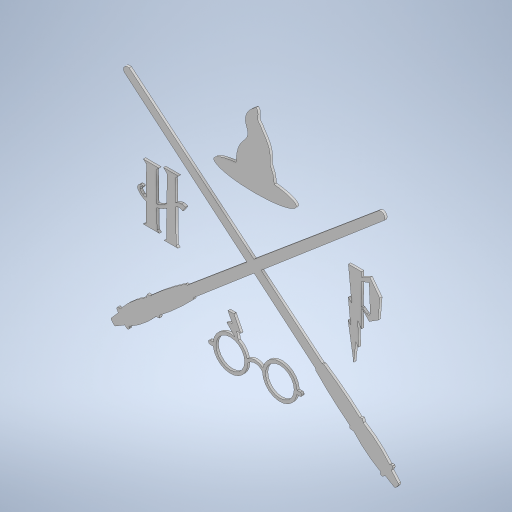
# Autodesk Inventor part: HP cross sign peices
Saved by Autodesk Inventor 2024 (Build 280153000, 153)
## iProperties
Created: 2023-06-06
Part Number: HP cross sign peices
Material: Generic
Document SubType Name: Modeling
Designer: newic
Density: 1 g/cm^3
Appearance: Default
Author: newic
Autodesk Inventor part; units mm, degrees
ref_plane "YZ Plane" through (0, 0, 0) normal (1, 0, 0) x (0, 1, 0)
ref_plane "XZ Plane" through (0, 0, 0) normal (0, 1, 0) x (-1, 0, 0)
ref_plane "XY Plane" through (0, 0, 0) normal (0, 0, 1) x (1, 0, 0)
sketch "Sketch1" plane through (0, 0, 0) normal (0, 0, 1) x (1, 0, 0)
  line L0 (50.8, 0) -> (355.6, 0)
  line L1 (406.4, 50.8) -> (406.4, 355.6)
  line L2 (355.6, 406.4) -> (50.8, 406.4)
  line L3 (0, 355.6) -> (0, 50.8)
  line L4 (-614.419348, 544.235047) -> (888.726493, 544.235047) construction
  line L5 (888.726493, 544.235047) -> (888.726493, -583.124441) construction
  line L6 (888.726493, -583.124441) -> (-614.419348, -583.124441) construction
  line L7 (-614.419348, -583.124441) -> (-614.419348, 544.235047) construction
  line L8 (6.363818, 43.79595) -> (9.763503, 39.85729)
  line L9 (12.196347, 39.474947) -> (24.470176, 46.948616)
  line L10 (24.470176, 46.948616) -> (27.553601, 44.522314)
  line L11 (29.72239, 44.392306) -> (30.075019, 44.607026)
  line L12 (30.938043, 46.672901) -> (30.552839, 48.300319)
  arc A0 (30.552839, 48.300319) -> (68.057484, 78.865401) centre (-37.470935, 170.060789) ccw
  arc A1 (68.057484, 78.865401) -> (72.898915, 79.406809) centre (69.41099, 88.679409) ccw
  arc A2 (72.898915, 79.406809) -> (72.898915, 82.717894) centre (67.457972, 81.062352) ccw
  arc A3 (72.898915, 82.717894) -> (119.938243, 125.239443) centre (-186.405748, 416.852181) ccw
  arc A4 (119.938243, 125.239443) -> (119.938243, 127.366674) centre (115.200777, 126.303058) ccw
  arc A5 (383.588883, 351.74213) -> (376.499139, 359.921937) centre (378.691736, 354.659966) ccw
  line L13 (6.368301, 46.290626) -> (15.835186, 57.178989)
  line L14 (15.835186, 57.178989) -> (13.961148, 60.626079)
  line L15 (14.197196, 62.7859) -> (14.468084, 63.097463)
  line L16 (16.64955, 63.601304) -> (18.189169, 62.948274)
  arc A6 (54.618428, 94.787427) -> (18.189169, 62.948274) centre (126.797058, -24.556995) ccw
  arc A7 (55.965181, 99.469183) -> (54.618428, 94.787427) centre (64.52036, 94.473621) ccw
  arc A8 (59.229243, 98.913144) -> (55.965181, 99.469183) centre (56.683501, 93.827491) ccw
  arc A9 (109.046352, 138.143695) -> (59.229243, 98.913144) centre (345.072656, -212.820994) ccw
  arc A10 (111.143373, 137.786464) -> (109.046352, 138.143695) centre (109.299288, 133.294893) ccw
  arc A11 (383.535154, 351.737832) -> (376.60786, 360.012951) centre (378.661869, 354.695351) ccw
  arc A12 (27.553601, 44.522314) -> (29.72239, 44.392306) centre (28.731635, 46.019399) ccw
  arc A13 (9.763503, 39.85729) -> (12.196347, 39.474947) centre (11.205592, 41.10204) ccw
  arc A14 (6.368301, 46.290626) -> (6.363818, 43.79595) centre (7.805907, 45.0407) ccw
  arc A15 (14.197196, 62.7859) -> (13.961148, 60.626079) centre (15.634801, 61.535974) ccw
  arc A16 (16.64955, 63.601304) -> (14.468084, 63.097463) centre (15.90569, 61.847537) ccw
  arc A17 (30.075019, 44.607026) -> (30.938043, 46.672901) centre (29.084264, 46.234118) ccw
  line L17 (399.519466, 39.849724) -> (402.80794, 43.881702)
  line L18 (402.762015, 46.343978) -> (393.27056, 57.133552)
  line L19 (393.27056, 57.133552) -> (395.12457, 60.591456)
  line L20 (394.875997, 62.749871) -> (394.603305, 63.059857)
  line L21 (392.418953, 63.551035) -> (390.883149, 62.889085)
  arc A18 (390.883149, 62.889085) -> (354.269806, 94.516378) centre (282.784699, -25.244739) ccw
  arc A19 (354.269806, 94.516378) -> (352.895917, 99.190243) centre (344.369861, 94.145137) ccw
  arc A20 (352.895917, 99.190243) -> (349.635135, 98.615279) centre (352.210336, 93.544479) ccw
  arc A21 (349.635135, 98.615279) -> (299.591291, 137.556184) centre (65.604881, -214.771773) ccw
  arc A22 (299.591291, 137.556184) -> (297.496377, 137.186795) centre (299.366486, 132.705996) ccw
  arc A23 (340.923339, 78.516662) -> (378.604658, 48.169656) centre (445.920964, 170.322678) ccw
  line L22 (384.69506, 46.853261) -> (381.625761, 44.409113)
  line L23 (397.061911, 39.420944) -> (384.69506, 46.853261)
  line L24 (379.457764, 44.266526) -> (379.103895, 44.479196)
  line L25 (378.228901, 46.54003) -> (378.604658, 48.169656)
  arc A24 (336.078849, 79.029976) -> (340.923339, 78.516662) centre (339.512925, 88.322652) ccw
  arc A25 (336.059641, 82.341005) -> (336.078849, 79.029976) centre (341.510096, 80.717053) ccw
  arc A26 (288.77444, 124.588966) -> (336.059641, 82.341005) centre (593.42165, 417.973879) ccw
  arc A27 (288.7621, 126.716161) -> (288.77444, 124.588966) centre (293.505656, 125.680045) ccw
  arc A28 (30.856483, 357.779219) -> (23.814309, 349.558422) centre (28.694447, 352.504618) ccw
  arc A29 (395.12457, 60.591456) -> (394.875997, 62.749871) centre (393.445666, 61.491627) ccw
  arc A30 (402.80794, 43.881702) -> (402.762015, 46.343978) centre (401.331684, 45.085734) ccw
  arc A31 (397.061911, 39.420944) -> (399.519466, 39.849724) centre (398.04321, 41.053756) ccw
  arc A32 (379.457764, 44.266526) -> (381.625761, 44.409113) centre (380.439063, 45.899338) ccw
  arc A33 (378.228901, 46.54003) -> (379.103895, 44.479196) centre (380.085194, 46.112009) ccw
  arc A34 (394.603305, 63.059857) -> (392.418953, 63.551035) centre (393.172975, 61.801613) ccw
  line L26 (401.147574, 41.845938) -> (389.574066, 107.482563) construction
  line L27 (321.553196, 108.082514) -> (389.468279, 108.082514) construction
  circle A35 centre (170.75121, 85.859958) radius 19.77729
  circle A36 centre (239.095683, 86.367375) radius 19.77729
  arc A37 (215.16651, 86.367375) -> (194.675003, 86.367375) centre (204.920756, 78.710251) ccw
  arc A38 (215.689784, 91.344244) -> (194.061536, 91.266807) centre (204.920756, 78.710251) ccw
  line L28 (269.404649, 85.988013) -> (269.404649, 84.655093)
  line L29 (140.68774, 84.655093) -> (140.68774, 85.988013)
  line L30 (267.499649, 82.750093) -> (262.749871, 82.750093)
  line L31 (147.024978, 82.750093) -> (142.59274, 82.750093)
  line L32 (142.59274, 87.893013) -> (146.908559, 87.893013)
  line L33 (262.976172, 87.893013) -> (267.499649, 87.893013)
  arc A39 (142.59274, 87.893013) -> (140.68774, 85.988013) centre (142.59274, 85.988013) ccw
  arc A40 (140.68774, 84.655093) -> (142.59274, 82.750093) centre (142.59274, 84.655093) ccw
  arc A41 (267.499649, 82.750093) -> (269.404649, 84.655093) centre (267.499649, 84.655093) ccw
  arc A42 (269.404649, 85.988013) -> (267.499649, 87.893013) centre (267.499649, 85.988013) ccw
  line L34 (176.805781, 109.010498) -> (165.933338, 120.455956)
  line L35 (173.368384, 123.688879) -> (167.378721, 135.467811)
  line L36 (167.60513, 135.836942) -> (175.47758, 135.836942)
  line L37 (175.703989, 135.698072) -> (185.025768, 117.366391)
  line L38 (184.799359, 116.99726) -> (179.672528, 116.99726)
  line L39 (179.426041, 116.681942) -> (181.815289, 107.077674)
  line L40 (166.035192, 120.871189) -> (173.224277, 123.333452)
  arc A43 (166.035192, 120.871189) -> (165.933338, 120.455956) centre (166.117494, 120.630892) ccw
  arc A44 (179.672528, 116.99726) -> (179.426041, 116.681942) centre (179.672528, 116.74326) ccw
  arc A45 (173.224277, 123.333452) -> (173.368384, 123.688879) centre (173.141975, 123.573749) ccw
  arc A46 (184.799359, 116.99726) -> (185.025768, 117.366391) centre (184.799359, 117.25126) ccw
  arc A47 (175.703989, 135.698072) -> (175.47758, 135.836942) centre (175.47758, 135.582942) ccw
  arc A48 (167.60513, 135.836942) -> (167.378721, 135.467811) centre (167.60513, 135.582942) ccw
  line L41 (79.178486, 175.528718) -> (98.216612, 175.528718)
  line L42 (98.216612, 175.528718) -> (95.757723, 177.666599)
  line L43 (79.178486, 175.528718) -> (82.322522, 178.515348)
  line L44 (83.401566, 257.118075) -> (78.414715, 262.36775)
  line L45 (78.414715, 262.36775) -> (99.063012, 262.36775)
  line L46 (99.063012, 262.36775) -> (94.659721, 258.18491)
  arc A49 (104.876764, 223.458347) -> (95.13125, 223.606943) centre (99.925457, 218.381083) ccw
  arc A50 (103.246066, 231.262323) -> (95.066939, 228.322925) centre (103.717194, 217.10211) ccw
  arc A51 (109.046352, 230.12172) -> (103.246066, 231.262323) centre (102.604733, 212.682614) ccw
  line L47 (104.876764, 223.458347) -> (109.046352, 230.12172)
  arc A52 (68.934077, 213.993149) -> (82.910758, 221.36528) centre (58.833092, 250.078534) ccw
  arc A53 (69.00456, 209.415023) -> (82.833167, 215.713199) centre (58.833092, 250.078534) ccw
  line L48 (68.309171, 254.582837) -> (71.925781, 258.465439)
  line L49 (71.925781, 258.465439) -> (50.439964, 258.597904)
  line L50 (50.439964, 258.597904) -> (54.618428, 254.705701)
  line L51 (54.180223, 183.62886) -> (50.217049, 180.722268)
  line L52 (50.217049, 180.722268) -> (72.473079, 180.585054)
  line L53 (72.473079, 180.585054) -> (69.41099, 183.016097)
  arc A54 (49.876677, 216.000145) -> (54.372837, 214.870815) centre (53.327561, 220.224164) ccw
  arc A55 (46.111078, 220.518863) -> (49.876677, 216.000145) centre (54.303486, 223.517512) ccw
  arc A56 (46.539208, 223.606943) -> (46.111078, 220.518863) centre (48.44907, 221.768443) ccw
  arc A57 (49.303504, 223.746898) -> (46.539208, 223.606943) centre (48.03713, 221.390233) ccw
  arc A58 (50.495329, 225.859285) -> (49.303504, 223.746898) centre (51.842309, 223.706896) ccw
  arc A59 (50.495329, 225.859285) -> (46.539208, 226.329877) centre (48.121838, 222.770318) ccw
  arc A60 (46.539208, 226.329877) -> (42.629235, 222.901423) centre (48.780718, 219.829765) ccw
  arc A61 (42.629235, 222.901423) -> (44.2476, 216.93411) centre (48.159437, 221.198131) ccw
  arc A62 (44.2476, 216.93411) -> (54.343434, 210.101637) centre (58.241765, 226.737074) ccw
  ellipse E0 centre (204.861319, 307.520258) end of major axis (261.987782, 307.520258) minor radius 12.590113 (178.424158, 318.681034) -> (231.29848, 318.681034) ccw
  spline S0 degree 4 poles (178.424158, 318.681034) (179.286467, 323.908779) (178.746893, 329.903111) (181.705459, 341.161729) (188.374596, 349.276888) (192.595103, 353.973206) (195.221019, 358.516301) (195.296154, 364.688161) (192.664089, 369.267258) (190.583011, 375.858216) (192.831333, 385.567134) (196.944916, 391.686323) (204.688734, 396.950297) (206.423918, 398.265857) knots 0 0 0 0 0 0.21195074 0.29434202 0.37160428 0.44319933 0.51142961 0.58048484 0.65260868 0.72741885 0.80713657 1 1 1 1 1
  spline S1 degree 4 poles (231.29848, 318.681034) (230.812293, 323.383734) (230.310579, 325.948758) (229.967534, 332.297352) (225.164417, 337.865291) (225.794617, 343.609489) (225.873041, 348.569917) (225.596308, 353.136069) (224.268791, 359.169129) (219.906128, 368.536889) (215.480963, 372.873287) (212.6971, 379.704121) (210.084613, 381.955148) (208.358926, 383.728321) (209.16421, 389.030713) (208.726826, 393.481301) (209.350832, 395.663281) (206.387951, 397.79334) (206.423918, 398.265857) knots 0 0 0 0 0 0.14868292 0.20666124 0.26562711 0.32344479 0.38253037 0.44758088 0.5167693 0.58902303 0.65607066 0.71151816 0.76312054 0.81115478 0.85814688 0.90611656 1 1 1 1 1
  line L54 (344.02064, 186.46558) -> (341.227275, 160.617354)
  line L55 (341.227275, 160.617354) -> (333.409452, 207.367115)
  line L56 (333.409452, 207.367115) -> (336.992659, 203.165326)
  line L57 (336.992659, 203.165326) -> (333.673251, 234.780696)
  line L58 (333.673251, 234.780696) -> (338.519545, 230.387183)
  line L59 (338.519545, 230.387183) -> (333.891431, 274.467202)
  line L60 (333.891431, 274.467202) -> (352.210336, 274.467202)
  line L61 (352.210336, 274.467202) -> (352.210336, 267.640425)
  line L62 (352.210336, 267.640425) -> (363.576578, 273.420233)
  line L63 (363.576578, 273.420233) -> (377.295, 255.343095)
  line L64 (377.295, 255.343095) -> (374.999674, 227.922054)
  line L65 (374.999674, 227.922054) -> (362.58525, 220.224164)
  line L66 (362.58525, 220.224164) -> (353.775486, 229.691563)
  line L67 (353.775486, 229.691563) -> (351.68678, 229.917285)
  line L68 (351.68678, 229.917285) -> (352.014132, 205.911995)
  line L69 (352.014132, 205.911995) -> (346.906345, 213.168267)
  line L70 (346.906345, 213.168267) -> (347.892244, 181.925607)
  line L71 (347.892244, 181.925607) -> (344.02064, 186.46558)
  line L72 (351.658839, 231.966214) -> (353.63723, 231.752414)
  line L73 (353.63723, 231.752414) -> (359.583199, 227.519206)
  line L74 (359.583199, 227.519206) -> (362.173085, 227.109648)
  line L75 (362.173085, 227.109648) -> (364.249648, 230.605551)
  line L76 (364.249648, 230.605551) -> (362.58525, 266.672272)
  line L77 (362.58525, 266.672272) -> (352.014132, 262.742303)
  line L78 (352.014132, 262.742303) -> (351.658839, 231.966214)
  line L79 (94.659721, 258.18491) -> (95.066939, 228.322925)
  line L80 (95.13125, 223.606943) -> (95.757723, 177.666599)
  line L81 (82.322522, 178.515348) -> (82.833167, 215.713199)
  line L82 (82.910758, 221.36528) -> (83.401566, 257.118075)
  line L83 (69.41099, 183.016097) -> (69.00456, 209.415023)
  line L84 (68.934077, 213.993149) -> (68.309171, 254.582837)
  line L85 (54.618428, 254.705701) -> (54.372837, 214.870815)
  line L86 (54.343434, 210.101637) -> (54.180223, 183.62886)
  line L87 (288.7621, 126.716161) -> (203.469206, 198.4543)
  line L88 (193.5656, 206.784024) -> (23.814309, 349.558422)
  line L89 (111.143373, 137.786464) -> (193.5656, 206.784024)
  line L90 (203.409935, 215.024946) -> (376.60786, 360.012951)
  line L91 (297.496377, 137.186795) -> (213.313238, 206.831897)
  line L92 (203.409935, 215.024946) -> (30.747236, 357.8696)
  line L93 (119.938243, 127.366674) -> (203.469206, 198.4543)
  line L94 (213.313238, 206.831897) -> (383.588883, 351.74213)
  arc A63 (147.024978, 82.750093) -> (194.675003, 86.367375) centre (170.75121, 85.859958) ccw
  arc A64 (194.061536, 91.266807) -> (181.815289, 107.077674) centre (170.75121, 85.859958) ccw
  arc A65 (176.805781, 109.010498) -> (146.908559, 87.893013) centre (170.75121, 85.859958) ccw
  arc A66 (215.16651, 86.367375) -> (262.749871, 82.750093) centre (239.095683, 86.367375) ccw
  arc A67 (262.976172, 87.893013) -> (215.689784, 91.344244) centre (239.095683, 86.367375) ccw
  arc A68 (0, 50.8) -> (50.8, 0) centre (50.8, 50.8) ccw
  arc A69 (355.6, 0) -> (406.4, 50.8) centre (355.6, 50.8) ccw
  arc A70 (406.4, 355.6) -> (355.6, 406.4) centre (355.6, 355.6) ccw
  arc A71 (50.8, 406.4) -> (0, 355.6) centre (50.8, 355.6) ccw
  point P0 (0, 0)
  point P1 (406.4, 406.4)
  point P2 (406.4, 0)
  point P3 (0, 406.4)
  point P4 (0, 51.168666)
  point P5 (10.817977, 38.635643)
  point P6 (28.59287, 43.704529)
  point P7 (31.256714, 45.326573)
  point P8 (5.347622, 45.116689)
  point P9 (13.329503, 61.787921)
  point P10 (15.375857, 64.141541)
  point P11 (179.198193, 326.398969)
  point P12 (180.643488, 334.841283)
  point P13 (184.294349, 343.588045)
  point P14 (188.857454, 349.748318)
  point P15 (192.58381, 354.387156)
  point P16 (194.713184, 358.874049)
  point P17 (194.789154, 364.197382)
  point P18 (192.963469, 369.215634)
  point P19 (191.366125, 375.527158)
  point P20 (192.431013, 382.448126)
  point P21 (195.777407, 388.760699)
  point P22 (202.089525, 394.996718)
  point P23 (230.558885, 324.790873)
  point P24 (229.864918, 328.854993)
  point P25 (228.278944, 333.514177)
  point P26 (225.999136, 338.173488)
  point P27 (225.701673, 343.625386)
  point P28 (225.800615, 348.383168)
  point P29 (225.50309, 352.546274)
  point P30 (224.115391, 358.494162)
  point P31 (219.555898, 368.011288)
  point P32 (215.095419, 374.554337)
  point P33 (211.923531, 380.006823)
  point P34 (210.040123, 382.088572)
  point P35 (208.949651, 383.971886)
  point P36 (208.949495, 388.927986)
  point P37 (208.949275, 392.793548)
  point P38 (208.651649, 395.073014)
  point P39 (207.164723, 397.25383)
  dimension "d0" = 406.4
  dimension "d1" = 406.4
  dimension "d37" = 1.905
  dimension "d38" = 1.905
  dimension "d40" = 1.905
  dimension "d41" = 1.905
  dimension "d43" = 1.905
  dimension "d44" = 1.905
  dimension "d45" = 1.905
  dimension "d46" = 1.905
  dimension "d62" = 3.81
  dimension "d69" = 1.905
  dimension "d73" = 0.254
  dimension "d80" = 50.8
  constraints: 182 end point, 141 point on circle, 72 centre point, 52 tangent, 27 point on line, 15 equal radius, 15 parallel, 9 horizontal, 7 perpendicular, 2 coincident, 41 other
  measures "d0" distance of point (0, 406.4) point (406.4, 406.4)
  measures "d1" distance of point (406.4, 406.4) point (406.4, 0)
  measures "d37" radius of A12
  measures "d38" radius of A13
  measures "d40" radius of A14
  measures "d41" radius of A15
  measures "d43" radius of A29
  measures "d44" radius of A30
  measures "d45" radius of A31
  measures "d46" radius of A32
  measures "d62" radial gap between concentric circles of A37 A38
  measures "d69" radius of A39
  measures "d73" radius of A43
  measures "d80" radius of A68
sketch "Sketch1 outline for Extrusion1" plane through (0, 0, 0) normal (0, 0, 1) x (1, 0, 0)
  arc A0 (267.499649, 82.750093) -> (269.404649, 84.655093) centre (267.499649, 84.655093) ccw
  line L0 (262.749871, 82.750093) -> (267.499649, 82.750093)
  line L1 (269.404649, 84.655093) -> (269.404649, 85.988013)
  arc A1 (215.16651, 86.367375) -> (262.749871, 82.750093) centre (239.095683, 86.367375) ccw
  arc A2 (269.404649, 85.988013) -> (267.499649, 87.893013) centre (267.499649, 85.988013) ccw
  arc A3 (194.675003, 86.367375) -> (215.16651, 86.367375) centre (204.920756, 78.710251) cw
  line L2 (267.499649, 87.893013) -> (262.976172, 87.893013)
  arc A4 (147.024978, 82.750093) -> (194.675003, 86.367375) centre (170.75121, 85.859958) ccw
  arc A5 (262.976172, 87.893013) -> (215.689784, 91.344244) centre (239.095683, 86.367375) ccw
  line L3 (142.59274, 82.750093) -> (147.024978, 82.750093)
  arc A6 (215.689784, 91.344244) -> (194.061536, 91.266807) centre (204.920756, 78.710251) ccw
  arc A7 (140.68774, 84.655093) -> (142.59274, 82.750093) centre (142.59274, 84.655093) ccw
  arc A8 (194.061536, 91.266807) -> (181.815289, 107.077674) centre (170.75121, 85.859958) ccw
  line L4 (140.68774, 85.988013) -> (140.68774, 84.655093)
  line L5 (181.815289, 107.077674) -> (179.426041, 116.681942)
  arc A9 (142.59274, 87.893013) -> (140.68774, 85.988013) centre (142.59274, 85.988013) ccw
  arc A10 (179.426041, 116.681942) -> (179.672528, 116.99726) centre (179.672528, 116.74326) cw
  line L6 (146.908559, 87.893013) -> (142.59274, 87.893013)
  line L7 (179.672528, 116.99726) -> (184.799359, 116.99726)
  arc A11 (176.805781, 109.010498) -> (146.908559, 87.893013) centre (170.75121, 85.859958) ccw
  arc A12 (184.799359, 116.99726) -> (185.025768, 117.366391) centre (184.799359, 117.25126) ccw
  line L8 (165.933338, 120.455956) -> (176.805781, 109.010498)
  line L9 (185.025768, 117.366391) -> (175.703989, 135.698072)
  arc A13 (166.035192, 120.871189) -> (165.933338, 120.455956) centre (166.117494, 120.630892) ccw
  arc A14 (175.703989, 135.698072) -> (175.47758, 135.836942) centre (175.47758, 135.582942) ccw
  line L10 (173.224277, 123.333452) -> (166.035192, 120.871189)
  line L11 (175.47758, 135.836942) -> (167.60513, 135.836942)
  arc A15 (173.368384, 123.688879) -> (173.224277, 123.333452) centre (173.141975, 123.573749) cw
  arc A16 (167.60513, 135.836942) -> (167.378721, 135.467811) centre (167.60513, 135.582942) ccw
  line L12 (167.378721, 135.467811) -> (173.368384, 123.688879)
  circle A17 centre (170.75121, 85.859958) radius 19.77729
  circle A18 centre (239.095683, 86.367375) radius 19.77729
  line L13 (344.02064, 186.46558) -> (347.892244, 181.925607)
  line L14 (341.227275, 160.617354) -> (344.02064, 186.46558)
  line L15 (347.892244, 181.925607) -> (346.906345, 213.168267)
  line L16 (333.409452, 207.367115) -> (341.227275, 160.617354)
  line L17 (346.906345, 213.168267) -> (352.014132, 205.911995)
  line L18 (336.992659, 203.165326) -> (333.409452, 207.367115)
  line L19 (352.014132, 205.911995) -> (351.68678, 229.917285)
  line L20 (333.673251, 234.780696) -> (336.992659, 203.165326)
  line L21 (351.68678, 229.917285) -> (353.775486, 229.691563)
  line L22 (338.519545, 230.387183) -> (333.673251, 234.780696)
  line L23 (353.775486, 229.691563) -> (362.58525, 220.224164)
  line L24 (333.891431, 274.467202) -> (338.519545, 230.387183)
  line L25 (362.58525, 220.224164) -> (374.999674, 227.922054)
  line L26 (352.210336, 274.467202) -> (333.891431, 274.467202)
  line L27 (374.999674, 227.922054) -> (377.295, 255.343095)
  line L28 (352.210336, 267.640425) -> (352.210336, 274.467202)
  line L29 (377.295, 255.343095) -> (363.576578, 273.420233)
  line L30 (363.576578, 273.420233) -> (352.210336, 267.640425)
  line L31 (351.658839, 231.966214) -> (352.014132, 262.742303)
  line L32 (353.63723, 231.752414) -> (351.658839, 231.966214)
  line L33 (359.583199, 227.519206) -> (353.63723, 231.752414)
  line L34 (362.173085, 227.109648) -> (359.583199, 227.519206)
  line L35 (364.249648, 230.605551) -> (362.173085, 227.109648)
  line L36 (362.58525, 266.672272) -> (364.249648, 230.605551)
  line L37 (352.014132, 262.742303) -> (362.58525, 266.672272)
  spline S0 degree 2 poles (178.424158, 318.681034) (116.307715, 311.534236) (160.584517, 299.56482) (204.861319, 287.595404) (249.138121, 299.56482) (293.414923, 311.534236) (231.29848, 318.681034) knots 0 0 0 0.33333333 0.33333333 0.66666667 0.66666667 1 1 1 weights 1 0.6318798 1 0.6318798 1 0.6318798 1
  spline S1 degree 4 poles (178.424158, 318.681034) (179.286467, 323.908779) (178.746893, 329.903111) (181.705459, 341.161729) (188.374596, 349.276888) (192.595103, 353.973206) (195.221019, 358.516301) (195.296154, 364.688161) (192.664089, 369.267258) (190.583011, 375.858216) (192.831333, 385.567134) (196.944916, 391.686323) (204.688734, 396.950297) (206.423918, 398.265857) knots 0 0 0 0 0 0.21195074 0.29434202 0.37160428 0.44319933 0.51142961 0.58048484 0.65260868 0.72741885 0.80713657 1 1 1 1 1
  spline S2 degree 4 poles (231.29848, 318.681034) (230.812293, 323.383734) (230.310579, 325.948758) (229.967534, 332.297352) (225.164417, 337.865291) (225.794617, 343.609489) (225.873041, 348.569917) (225.596308, 353.136069) (224.268791, 359.169129) (219.906128, 368.536889) (215.480963, 372.873287) (212.6971, 379.704121) (210.084613, 381.955148) (208.358926, 383.728321) (209.16421, 389.030713) (208.726826, 393.481301) (209.350832, 395.663281) (206.387951, 397.79334) (206.423918, 398.265857) knots 0 0 0 0 0 0.14868292 0.20666124 0.26562711 0.32344479 0.38253037 0.44758088 0.5167693 0.58902303 0.65607066 0.71151816 0.76312054 0.81115478 0.85814688 0.90611656 1 1 1 1 1
  line L38 (82.322522, 178.515348) -> (79.178486, 175.528718)
  line L39 (82.833167, 215.713199) -> (82.322522, 178.515348)
  arc A19 (69.00456, 209.415023) -> (82.833167, 215.713199) centre (58.833092, 250.078534) ccw
  line L40 (69.41099, 183.016097) -> (69.00456, 209.415023)
  line L41 (72.473079, 180.585054) -> (69.41099, 183.016097)
  line L42 (50.217049, 180.722268) -> (72.473079, 180.585054)
  line L43 (54.180223, 183.62886) -> (50.217049, 180.722268)
  line L44 (54.343434, 210.101637) -> (54.180223, 183.62886)
  arc A20 (44.2476, 216.93411) -> (54.343434, 210.101637) centre (58.241765, 226.737074) ccw
  arc A21 (42.629235, 222.901423) -> (44.2476, 216.93411) centre (48.159437, 221.198131) ccw
  arc A22 (46.539208, 226.329877) -> (42.629235, 222.901423) centre (48.780718, 219.829765) ccw
  arc A23 (50.495329, 225.859285) -> (46.539208, 226.329877) centre (48.121838, 222.770318) ccw
  arc A24 (49.303504, 223.746898) -> (50.495329, 225.859285) centre (51.842309, 223.706896) cw
  arc A25 (46.539208, 223.606943) -> (49.303504, 223.746898) centre (48.03713, 221.390233) cw
  arc A26 (46.111078, 220.518863) -> (46.539208, 223.606943) centre (48.44907, 221.768443) cw
  arc A27 (49.876677, 216.000145) -> (46.111078, 220.518863) centre (54.303486, 223.517512) cw
  arc A28 (54.372837, 214.870815) -> (49.876677, 216.000145) centre (53.327561, 220.224164) cw
  line L45 (54.618428, 254.705701) -> (54.372837, 214.870815)
  line L46 (50.439964, 258.597904) -> (54.618428, 254.705701)
  line L47 (71.925781, 258.465439) -> (50.439964, 258.597904)
  line L48 (68.309171, 254.582837) -> (71.925781, 258.465439)
  line L49 (68.934077, 213.993149) -> (68.309171, 254.582837)
  arc A29 (82.910758, 221.36528) -> (68.934077, 213.993149) centre (58.833092, 250.078534) cw
  line L50 (83.401566, 257.118075) -> (82.910758, 221.36528)
  line L51 (78.414715, 262.36775) -> (83.401566, 257.118075)
  line L52 (99.063012, 262.36775) -> (78.414715, 262.36775)
  line L53 (94.659721, 258.18491) -> (99.063012, 262.36775)
  line L54 (95.066939, 228.322925) -> (94.659721, 258.18491)
  arc A30 (103.246066, 231.262323) -> (95.066939, 228.322925) centre (103.717194, 217.10211) ccw
  arc A31 (109.046352, 230.12172) -> (103.246066, 231.262323) centre (102.604733, 212.682614) ccw
  line L55 (104.876764, 223.458347) -> (109.046352, 230.12172)
  arc A32 (95.13125, 223.606943) -> (104.876764, 223.458347) centre (99.925457, 218.381083) cw
  line L56 (95.757723, 177.666599) -> (95.13125, 223.606943)
  line L57 (98.216612, 175.528718) -> (95.757723, 177.666599)
  line L58 (79.178486, 175.528718) -> (98.216612, 175.528718)
  line L59 (213.313238, 206.831897) -> (383.588883, 351.74213)
  line L60 (297.496377, 137.186795) -> (213.313238, 206.831897)
  arc A33 (299.591291, 137.556184) -> (297.496377, 137.186795) centre (299.366486, 132.705996) ccw
  arc A34 (349.635135, 98.615279) -> (299.591291, 137.556184) centre (65.604881, -214.771773) ccw
  arc A35 (352.895917, 99.190243) -> (349.635135, 98.615279) centre (352.210336, 93.544479) ccw
  arc A36 (354.269806, 94.516378) -> (352.895917, 99.190243) centre (344.369861, 94.145137) ccw
  arc A37 (390.883149, 62.889085) -> (354.269806, 94.516378) centre (282.784699, -25.244739) ccw
  line L61 (392.418953, 63.551035) -> (390.883149, 62.889085)
  arc A38 (394.603305, 63.059857) -> (392.418953, 63.551035) centre (393.172975, 61.801613) ccw
  line L62 (394.875997, 62.749871) -> (394.603305, 63.059857)
  arc A39 (395.12457, 60.591456) -> (394.875997, 62.749871) centre (393.445666, 61.491627) ccw
  line L63 (393.27056, 57.133552) -> (395.12457, 60.591456)
  line L64 (402.762015, 46.343978) -> (393.27056, 57.133552)
  arc A40 (402.80794, 43.881702) -> (402.762015, 46.343978) centre (401.331684, 45.085734) ccw
  line L65 (399.519466, 39.849724) -> (402.80794, 43.881702)
  arc A41 (397.061911, 39.420944) -> (399.519466, 39.849724) centre (398.04321, 41.053756) ccw
  line L66 (384.69506, 46.853261) -> (397.061911, 39.420944)
  line L67 (381.625761, 44.409113) -> (384.69506, 46.853261)
  arc A42 (379.457764, 44.266526) -> (381.625761, 44.409113) centre (380.439063, 45.899338) ccw
  line L68 (379.103895, 44.479196) -> (379.457764, 44.266526)
  arc A43 (378.228901, 46.54003) -> (379.103895, 44.479196) centre (380.085194, 46.112009) ccw
  line L69 (378.604658, 48.169656) -> (378.228901, 46.54003)
  arc A44 (340.923339, 78.516662) -> (378.604658, 48.169656) centre (445.920964, 170.322678) ccw
  arc A45 (336.078849, 79.029976) -> (340.923339, 78.516662) centre (339.512925, 88.322652) ccw
  arc A46 (336.059641, 82.341005) -> (336.078849, 79.029976) centre (341.510096, 80.717053) ccw
  arc A47 (288.77444, 124.588966) -> (336.059641, 82.341005) centre (593.42165, 417.973879) ccw
  arc A48 (288.7621, 126.716161) -> (288.77444, 124.588966) centre (293.505656, 125.680045) ccw
  line L70 (203.469206, 198.4543) -> (288.7621, 126.716161)
  line L71 (119.938243, 127.366674) -> (203.469206, 198.4543)
  arc A49 (119.938243, 125.239443) -> (119.938243, 127.366674) centre (115.200777, 126.303058) ccw
  arc A50 (72.898915, 82.717894) -> (119.938243, 125.239443) centre (-186.405748, 416.852181) ccw
  arc A51 (72.898915, 79.406809) -> (72.898915, 82.717894) centre (67.457972, 81.062352) ccw
  arc A52 (68.057484, 78.865401) -> (72.898915, 79.406809) centre (69.41099, 88.679409) ccw
  arc A53 (30.552839, 48.300319) -> (68.057484, 78.865401) centre (-37.470935, 170.060789) ccw
  line L72 (30.938043, 46.672901) -> (30.552839, 48.300319)
  arc A54 (30.075019, 44.607026) -> (30.938043, 46.672901) centre (29.084264, 46.234118) ccw
  line L73 (29.72239, 44.392306) -> (30.075019, 44.607026)
  arc A55 (27.553601, 44.522314) -> (29.72239, 44.392306) centre (28.731635, 46.019399) ccw
  line L74 (24.470176, 46.948616) -> (27.553601, 44.522314)
  line L75 (12.196347, 39.474947) -> (24.470176, 46.948616)
  arc A56 (9.763503, 39.85729) -> (12.196347, 39.474947) centre (11.205592, 41.10204) ccw
  line L76 (6.363818, 43.79595) -> (9.763503, 39.85729)
  arc A57 (6.368301, 46.290626) -> (6.363818, 43.79595) centre (7.805907, 45.0407) ccw
  line L77 (15.835186, 57.178989) -> (6.368301, 46.290626)
  line L78 (13.961148, 60.626079) -> (15.835186, 57.178989)
  arc A58 (14.197196, 62.7859) -> (13.961148, 60.626079) centre (15.634801, 61.535974) ccw
  line L79 (14.468084, 63.097463) -> (14.197196, 62.7859)
  arc A59 (16.64955, 63.601304) -> (14.468084, 63.097463) centre (15.90569, 61.847537) ccw
  line L80 (18.189169, 62.948274) -> (16.64955, 63.601304)
  arc A60 (54.618428, 94.787427) -> (18.189169, 62.948274) centre (126.797058, -24.556995) ccw
  arc A61 (55.965181, 99.469183) -> (54.618428, 94.787427) centre (64.52036, 94.473621) ccw
  arc A62 (59.229243, 98.913144) -> (55.965181, 99.469183) centre (56.683501, 93.827491) ccw
  arc A63 (109.046352, 138.143695) -> (59.229243, 98.913144) centre (345.072656, -212.820994) ccw
  arc A64 (111.143373, 137.786464) -> (109.046352, 138.143695) centre (109.299288, 133.294893) ccw
  line L81 (193.5656, 206.784024) -> (111.143373, 137.786464)
  line L82 (23.814309, 349.558422) -> (193.5656, 206.784024)
  arc A65 (30.856483, 357.779219) -> (23.814309, 349.558422) centre (28.694447, 352.504618) ccw
  line L83 (203.409935, 215.024946) -> (30.856483, 357.779219)
  line L84 (376.499139, 359.921937) -> (203.409935, 215.024946)
  arc A66 (383.588883, 351.74213) -> (376.499139, 359.921937) centre (378.691736, 354.659966) ccw
extrude "Extrusion1" add sketch "Sketch1 outline for Extrusion1" along normal blind 3.175
body "Solid1"
